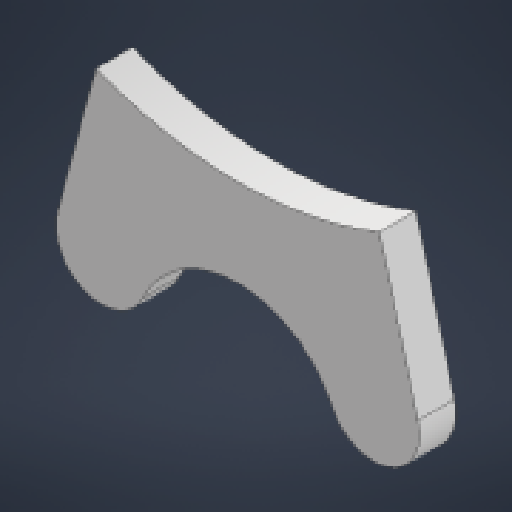
# Autodesk Inventor part: Gradient_positioner
Saved by Autodesk Inventor 2026.1 (Build 301233020, 233B)
## iProperties
Created: 2025-11-19
Part Number: Gradient_positioner
Material: Generic
Document SubType Name: Modeling
Designer: Carla Fernandez
Density: 1 g/cm^3
Appearance: Default
Author: Carla Fernandez
Autodesk Inventor part; units mm, degrees
ref_plane "YZ Plane" through (0, 0, 0) normal (1, 0, 0) x (0, 1, 0)
ref_plane "XY Plane" through (0, 0, 0) normal (0, 0, 1) x (1, 0, 0)
sketch "Sketch1" plane through (0, 0, 0) normal (0, 0, 1) x (1, 0, 0)
  arc A0 (-36.491, -107.2085) -> (-22.6527, -112.7232) centre (-29.2466, -109.1496) ccw
  arc A1 (-28.7685, -78.3877) -> (28.7685, -78.3877) centre (0, 0) ccw
  line L0 (0, 0) -> (0, -147.6951) construction
  line L1 (0, 0) -> (-29.2466, -109.1496) construction
  line L2 (-36.491, -107.2085) -> (-28.7685, -78.3877)
  arc A2 (0, -99.2345) -> (-22.6527, -112.7232) centre (0, -125) ccw
  arc A3 (22.6527, -112.7232) -> (36.491, -107.2085) centre (29.2466, -109.1496) ccw
  line L3 (36.491, -107.2085) -> (28.7685, -78.3877)
  arc A4 (22.6527, -112.7232) -> (0, -99.2345) centre (0, -125) ccw
  dimension "d0" = 167
  dimension "d1" = 15
  dimension "d2" = 15
  dimension "d3" = 113
  dimension "d4" = 125
  constraints: 12 point on circle, 8 end point, 5 centre point, 5 symmetric about line, 4 point on line, 2 tangent, 1 coincident, 1 parallel, 1 vertical, 2 other
  measures "d0" diameter of A1
  measures "d1" diameter of A0
  measures "d2" angle of L0 L1
  measures "d3" distance of L1.end point (0, 0)
  measures "d4" distance of A2.centre point (0, 0)
extrude "Extrusion1" add sketch "Sketch1" along normal blind 6
sketch "Sketch2" plane through (0, 0, 6) normal (0, 0, 1) x (1, 0, 0)
  line L0 (-29.2466, -109.1496) -> (0, 0) construction
  line L1 (0, 0) -> (29.2466, -109.1496) construction
  line L2 (0, 0) -> (0, -137.2486) construction
  dimension "d14" = 15
  dimension "d15" = 15
  dimension "d16" = 113
  dimension "d17" = 113
  constraints: 6 end point, 1 vertical
  measures "d14" angle of L2 L0
  measures "d15" angle of L1 L2
  measures "d16" distance of L0.start L0.end
  measures "d17" distance of L0.end L1.end
hole "Hole1" at (-29.2466, -109.1496, 6) at (29.2466, -109.1496, 6) direction (0, 0, -1) diameter 4.5 end through all countersink diameter 9.4 countersink angle 90 clearance for "Countersunk Flat Head Screw DIN EN ISO 2009" size "M4" standard "DIN"
fillet "Fillet1" radius 5 2 edges at (-28.7685, -78.3877, 3) (28.7685, -78.3877, 3)
ref_plane "Work Plane1" through (-25.3112, -79.8033, 0) normal (0, 1, 0) x (-1, 0, 0)
sketch "Sketch3" plane through (-25.3112, -79.8033, 0) normal (0, 1, 0) x (-1, 0, 0)
  line L0 (11.1798, 0) -> (11.1798, 6) projected
  point P0 (-25.3112, 0)
  point P1 (-25.3112, 3)
  point P2 (11.1798, 3)
  constraints: 1 horizontal alignment, 1 midpoint, 1 vertical alignment
hole "Hole2" at (0, -79.8033, 3) direction (0, -1, 0) diameter 4 end through all
equation "\"d15\" = d14"
equation "\"d17\" = d16"
body "Solid1"
